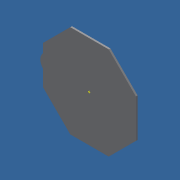
# Autodesk Inventor part: Oktagon_Deckel
Saved by Autodesk Inventor 2018.2 (Build 222227000, 227)
## iProperties
Created: 2018-10-01
Part Number: Oktagon_Deckel
Material: geeigneten Werkstoff auswählen !
Document SubType Name: Modeling
Designer: N.Grubert
Density: 0.001 g/cm^3
Appearance: Vorgabe
Fläche: 0 cm²
Gewicht: 0 g
Dateiname: P:\INVENTOR\Inventor 2018\Templates\ILT\Norm.ipt
Bez_eng: bolt
Bez_french: boulon
Author: N.Grubert
Autodesk Inventor part; units mm, degrees
ref_plane "YZ Plane" through (0, 0, 0) normal (1, 0, 0) x (0, 1, 0)
ref_plane "XZ Plane" through (0, 0, 0) normal (0, 1, 0) x (-1, 0, 0)
ref_plane "XY Plane" through (0, 0, 0) normal (0, 0, 1) x (1, 0, 0)
sketch "Skizze4" plane through (0, 0, 0) normal (0, 1, 0) x (-1, 0, 0)
  line L0 (27.9594, 67.5) -> (67.5, 27.9594)
  line L1 (67.5, 27.9594) -> (67.5, -27.9594)
  line L2 (67.5, -27.9594) -> (27.9594, -67.5)
  line L3 (27.9594, -67.5) -> (-27.9594, -67.5)
  line L4 (-27.9594, -67.5) -> (-67.5, -27.9594)
  line L5 (-67.5, -27.9594) -> (-67.5, 27.9594)
  line L6 (-67.5, 27.9594) -> (-27.9594, 67.5)
  line L7 (-27.9594, 67.5) -> (27.9594, 67.5)
  line L8 (0, -94.5) -> (0, 94.5) construction
  line L9 (94.5, 0) -> (-94.5, 0) construction
  point P0 (0, 0)
  point P1 (0, 0)
  dimension "d4" = 135
  constraints: 16 end point, 1 coincident, 18 other
  measures "d4" distance between parallel lines of L3 L7
extrude "Extrusion2" add sketch "Skizze4" along normal blind 2.5
sketch "Skizze5" plane through (0, 2.5, 0) normal (0, 1, 0) x (1, 0, 0)
  line L0 (21.7462, 52.5) -> (-21.7462, 52.5) projected
  line L1 (-21.7462, 52.5) -> (-52.5, 21.7462) projected
  line L2 (-52.5, 21.7462) -> (-52.5, -21.7462) projected
  line L3 (-52.5, -21.7462) -> (-21.7462, -52.5) projected
  line L4 (-21.7462, -52.5) -> (21.7462, -52.5) projected
  line L5 (21.7462, -52.5) -> (52.5, -21.7462) projected
  line L6 (52.5, -21.7462) -> (52.5, 21.7462) projected
  line L7 (52.5, 21.7462) -> (21.7462, 52.5) projected
  line L8 (22.7817, 55) -> (55, 22.7817) projected
  line L9 (55, 22.7817) -> (55, -22.7817) projected
  line L10 (55, -22.7817) -> (22.7817, -55) projected
  line L11 (22.7817, -55) -> (-22.7817, -55) projected
  line L12 (-22.7817, -55) -> (-55, -22.7817) projected
  line L13 (-55, -22.7817) -> (-55, 22.7817) projected
  line L14 (-55, 22.7817) -> (-22.7817, 55) projected
  line L15 (-22.7817, 55) -> (22.7817, 55) projected
  line L16 (-50, 20.7107) -> (-20.7107, 50)
  line L17 (-20.7107, 50) -> (20.7107, 50)
  line L18 (20.7107, 50) -> (50, 20.7107)
  line L19 (50, 20.7107) -> (50, -20.7107)
  line L20 (50, -20.7107) -> (20.7107, -50)
  line L21 (20.7107, -50) -> (-20.7107, -50)
  line L22 (-20.7107, -50) -> (-50, -20.7107)
  line L23 (-50, -20.7107) -> (-50, 20.7107)
  line L24 (52, -21.5391) -> (21.5391, -52)
  line L25 (21.5391, -52) -> (-21.5391, -52)
  line L26 (-21.5391, -52) -> (-52, -21.5391)
  line L27 (-52, -21.5391) -> (-52, 21.5391)
  line L28 (-52, 21.5391) -> (-21.5391, 52)
  line L29 (-21.5391, 52) -> (21.5391, 52)
  line L30 (21.5391, 52) -> (52, 21.5391)
  line L31 (52, 21.5391) -> (52, -21.5391)
  point P0 (0, 0)
  dimension "d7" = 2.5
  dimension "d19" = 0.5
  constraints: 32 end point, 14 other
  measures "d7" distance between parallel lines of L0 L17
  measures "d19" distance between parallel lines of L5 L24
extrude "Extrusion3" add sketch "Skizze5" along normal blind 3 contours L7 L6 L5 L4 L3 L2 L1 L0 | L24 L25 L26 L27 L28 L29 L30 L31
sketch "Skizze7" plane through (0, 0, 0) normal (0, -1, 0) x (1, 0, 0)
  line L0 (-27.9594, 67.5) -> (-67.5, 27.9594) construction
  line L1 (-67.5, 27.9594) -> (-67.5, -27.9594) construction
  line L2 (-67.5, -27.9594) -> (-27.9594, -67.5) construction
  line L3 (-27.9594, -67.5) -> (27.9594, -67.5) construction
  line L4 (27.9594, -67.5) -> (67.5, -27.9594) construction
  line L5 (67.5, -27.9594) -> (67.5, 27.9594) construction
  line L6 (67.5, 27.9594) -> (27.9594, 67.5) construction
  line L7 (27.9594, 67.5) -> (-27.9594, 67.5) construction
  line L8 (-67.5, 27.9594) -> (-67.5, -27.9594) projected
  arc A0 (-67.5, 14.8463) -> (-67.5, -4.7496) centre (-57.5, 5.0484) ccw
  point P0 (0, 0)
  dimension "d15" = 14
  dimension "d16" = 10
  constraints: 2 point on circle, 2 point on line, 1 centre point
  measures "d15" radius of A0
  measures "d16" distance from line of L1 A0.centre
extrude "Extrusion5" add sketch "Skizze7" against normal up to surface (2.5 mm away)
